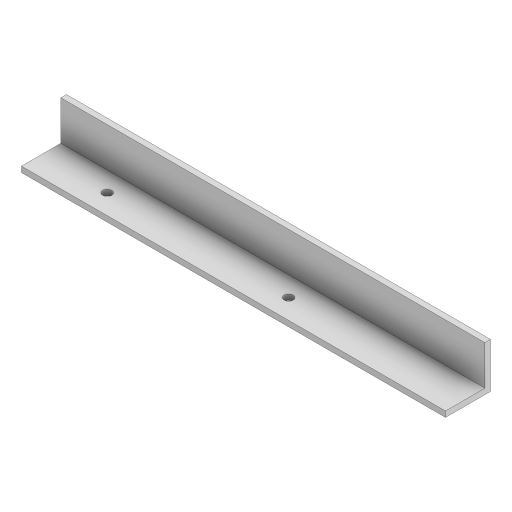
# Autodesk Inventor part: PERFIL_SOPORTE DEL MOTOR
Saved by Autodesk Inventor 2024 (Build 280153000, 153)
## iProperties
Created: 2024-06-24
Part Number: PERFIL_SOPORTE DEL MOTOR
Material: Generic
Document SubType Name: Modeling
Designer: Jhuliams
Density: 1 g/cm^3
Appearance: Default
Author: Jhuliams
Autodesk Inventor part; units mm, degrees
ref_plane "YZ Plane" through (0, 0, 0) normal (1, 0, 0) x (0, 1, 0)
ref_plane "XZ Plane" through (0, 0, 0) normal (0, 1, 0) x (-1, 0, 0)
ref_plane "XY Plane" through (0, 0, 0) normal (0, 0, 1) x (1, 0, 0)
sketch "Sketch1" plane through (0, 0, 0) normal (1, 0, 0) x (0, 1, 0)
  line L0 (0, 0) -> (25.4, 0)
  line L1 (25.4, 0) -> (25.4, 3.175)
  line L2 (25.4, 3.175) -> (0, 3.175)
  line L3 (0, 3.175) -> (0, 0)
  line L4 (0, 0) -> (3.175, 0)
  line L5 (3.175, 0) -> (3.175, 25.4)
  line L6 (3.175, 25.4) -> (0, 25.4)
  line L7 (0, 25.4) -> (0, 0)
  point P0 (3.175, 3.175)
  dimension "d0" = 25.4
  dimension "d1" = 3.175
  dimension "d2" = 3.175
  dimension "d3" = 25.4
  constraints: 16 end point, 4 parallel, 2 horizontal, 2 perpendicular
  measures "d0" distance of L2.end L1.end
  measures "d1" distance of L1.end L0.end
  measures "d2" distance of L6.end L5.end
  measures "d3" distance of L5.end L4.end
extrude "Extrusion1" add sketch "Sketch1" along normal blind 239
sketch "Sketch2" plane through (0, 3.175, 25.4) normal (0, 1, 0) x (1, 0, 0)
  line L0 (0, 22.225) -> (0, 0) projected
  line L1 (0, 0) -> (239, 0) projected
  line L2 (239, 22.225) -> (239, 0) projected
  line L3 (0, 22.225) -> (239, 22.225) projected
  line L4 (0, 11.1125) -> (74.5, 11.1125)
  line L5 (74.5, 11.1125) -> (139.5, 11.1125)
  circle A0 centre (37.25, 11.1125) radius 2.5
  circle A1 centre (139.5, 11.1125) radius 2.5
  point P0 (0, 25.4)
  dimension "d6" = 74.5
  dimension "d7" = 65
  dimension "d8" = 5
  dimension "d9" = 5
  constraints: 4 end point, 2 centre point, 2 horizontal, 2 midpoint, 1 coincident
  measures "d6" distance of L4.start L4.end
  measures "d7" distance of L4.end L5.end
  measures "d8" diameter of A0
  measures "d9" diameter of A1
extrude "Extrusion2" cut sketch "Sketch2" against normal blind 10 contours A0 L4 | L4 A0 | A1
body "Solid1"
